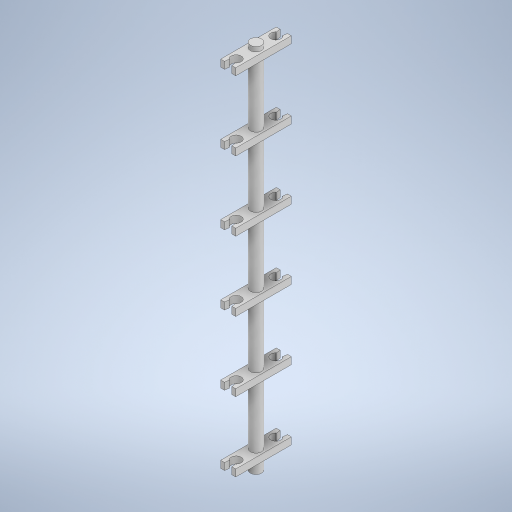
# Autodesk Inventor part: [3DP]double_bar
Saved by Autodesk Inventor 2024 (Build 280153000, 153)
## iProperties
Created: 2024-04-09
Part Number: [3DP]double_bar
Material: 一般
Document SubType Name: Modeling
Designer: USER
Density: 1 g/cm^3
Appearance: 預設
Author: USER
Autodesk Inventor part; units mm, degrees
ref_plane "YZ Plane" through (0, 0, 0) normal (1, 0, 0) x (0, 1, 0)
ref_plane "XZ Plane" through (0, 0, 0) normal (0, 1, 0) x (-1, 0, 0)
sketch "草圖1" plane through (0, 0, 0) normal (0, 1, 0) x (-1, 0, 0)
  circle A0 centre (0, 0) radius 2.45
  dimension "d0" = 4.9
  constraints: 1 centre point, 1 coincident
  measures "d0" diameter of A0
extrude "擠出1" add sketch "草圖1" along normal blind 160
ref_plane "工作平面1" through (0, 5, 0) normal (0, -1, 0) x (1, 0, 0)
sketch "草圖3" plane through (0, 5, 0) normal (0, -1, 0) x (1, 0, 0)
  circle A0 centre (0, 0) radius 2.45 projected
  circle A1 centre (0, 0) radius 3.25
  line L0 (3.25, 0) -> (-3.25, 0)
  line L1 (-3.25, 0) -> (-3.25, -12)
  line L2 (-3.25, -12) -> (3.25, -12)
  line L3 (3.25, -12) -> (3.25, 0)
  line L4 (1.6, -12) -> (-1.6, -12)
  line L5 (-1.6, -12) -> (-1.6, -7)
  line L6 (-1.6, -7) -> (1.6, -7)
  line L7 (1.6, -7) -> (1.6, -12)
  line L8 (1.55, -7) -> (-1.55, -7)
  line L9 (-1.55, -7) -> (-1.55, -10.1)
  line L10 (-1.55, -10.1) -> (1.55, -10.1)
  line L11 (1.55, -10.1) -> (1.55, -7)
  line L12 (1.55, -10.1) -> (1.35, -10.1)
  line L13 (1.35, -10.1) -> (1.6, -12)
  line L14 (-1.55, -10.1) -> (-1.35, -10.1)
  line L15 (-1.35, -10.1) -> (-1.6, -12)
  circle A2 centre (0, -8.55) radius 2.192
  line L16 (-3.25, 0) -> (-3.25, 12)
  line L17 (-3.25, 12) -> (3.25, 12)
  line L18 (3.25, 12) -> (3.25, 0)
  line L19 (1.6, 12) -> (-1.6, 12)
  line L20 (-1.6, 12) -> (-1.6, 7)
  line L21 (-1.6, 7) -> (1.6, 7)
  line L22 (1.6, 7) -> (1.6, 12)
  line L23 (1.55, 7) -> (-1.55, 7)
  line L24 (-1.55, 7) -> (-1.55, 10.1)
  line L25 (-1.55, 10.1) -> (1.55, 10.1)
  line L26 (1.55, 10.1) -> (1.55, 7)
  line L27 (1.55, 10.1) -> (1.35, 10.1)
  line L28 (1.35, 10.1) -> (1.6, 12)
  line L29 (-1.55, 10.1) -> (-1.35, 10.1)
  line L30 (-1.35, 10.1) -> (-1.6, 12)
  circle A3 centre (0, 8.55) radius 2.192
  point P0 (0, -12)
  point P1 (0, -12)
  point P2 (0, -7)
  point P3 (-1.55, -7)
  point P4 (1.55, -7)
  point P5 (-1.55, -8.55)
  point P6 (-1.3711, -10.2603)
  point P7 (1.3711, -10.2603)
  point P8 (0, 12)
  point P9 (0, 12)
  point P10 (0, 7)
  point P11 (-1.55, 8.55)
  point P12 (1.3711, 10.2603)
  point P13 (-1.3711, 10.2603)
  point P14 (0.9915, 3.095)
  point P15 (-0.9915, 3.095)
  point P16 (-1.55, 10.1)
  point P17 (-1.55, -10.1)
  point P18 (-1.55, -10.1)
  dimension "d17" = 6.5
  dimension "d9" = 12
  dimension "d11" = 5
  dimension "d12" = 3.2
  dimension "d13" = 3.1
  dimension "d14" = 3.1
  dimension "d15" = 0.2
  dimension "d16" = 0.2
  dimension "d18" = 6.5
  constraints: 62 end point, 17 symmetric about line, 8 midpoint, 6 parallel, 4 horizontal, 4 point on line, 3 perpendicular, 2 coincident, 2 vertical alignment, 1 horizontal alignment, 1 vertical, 9 other
  measures "d9" distance of L2.end L0.start
  measures "d11" distance of L6.end L4.start
  measures "d12" distance of L4.start L4.end
  measures "d13" distance of L9.end L10.end
  measures "d14" distance of L10.end L8.start
  measures "d15" distance of L10.end L12.end
  measures "d16" distance of L9.end L14.end
  measures "d18" distance of L1.end L2.end
extrude "擠出3" add sketch "草圖3" against normal blind 3 contours L0 A1 A0 | A0 L0 A1 | L3 L2 L7 A2 L6 L5 L1 A1 | A1 L16 L17 L20 A3 L21 L22 L18 | L13 A2 L7 | L22 A3 L28 | L5 A2 L15 | L30 A3 L20 | L13 L10 A2 | A3 L25 L28 | A2 L10 L15 | L30 L25 A3 | A2 L6 L7 | L22 L21 A3 | L5 L6 A2 | A3 L21 L20
pattern_linear "矩形陣列1" count 6 spacing 30 along (0, 1, 0) of "擠出3"
